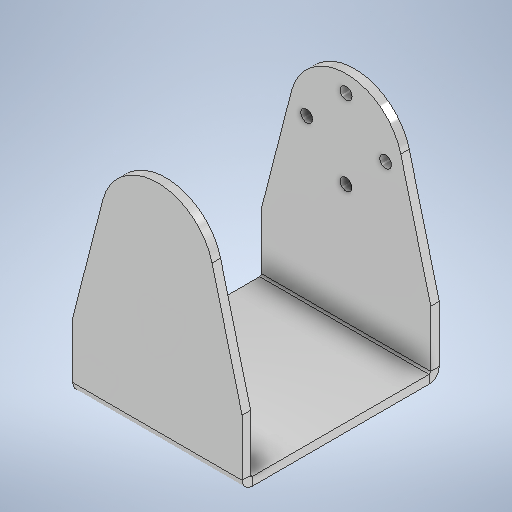
# Autodesk Inventor part: axis_12_bottom_frame(top)
Saved by Autodesk Inventor 2025.2 (Build 292293000, 293)
## iProperties
Created: 2025-05-04
Part Number: axis_12_bottom_frame(top)
Material: Aluminum 6061-AHC
Document SubType Name: Sheet Metal
Designer: User
Density: 2.7 g/cm^3
Sheet Metal Rule: Default_mm
Appearance: Aluminum - Dark
Author: User
Autodesk Inventor part; units mm, degrees
ref_plane "YZ Plane" through (0, 0, 0) normal (1, 0, 0) x (0, 1, 0)
ref_plane "XZ Plane" through (0, 0, 0) normal (0, 1, 0) x (-1, 0, 0)
ref_plane "XY Plane" through (0, 0, 0) normal (0, 0, 1) x (1, 0, 0)
sketch "Sketch1" plane through (0, 0, 0) normal (0, 1, 0) x (-1, 0, 0)
  line L0 (15, -15.965) -> (-15, -15.965)
  line L1 (-15, -15.965) -> (-15, 15.965)
  line L2 (-15, 15.965) -> (15, 15.965)
  line L3 (15, 15.965) -> (15, -15.965)
  point P0 (0, 0)
  dimension "d0" = 30
  dimension "d1" = 15
  dimension "d2" = 31.93
  dimension "d3" = 15.965
  measures "d0" distance of L0.start L0.end
  measures "d1" distance from line of point (0, 0) L3
  measures "d2" distance of L0.end L1.end
  measures "d3" distance from line of point (0, 0) L0
extrude "Plate1" add sketch "Sketch1" along normal blind 1.5
sketch "Sketch2" plane through (15, 0, 17.465) normal (0, 0, -1) x (-1, 0, 0)
  line L0 (30, 0) -> (0, 0)
  line L1 (0, 0) -> (0, 40)
  line L2 (0, 40) -> (30, 40)
  line L3 (30, 40) -> (30, 0)
  constraints: 8 end point
edge flange "Flange1" height 40 angle 90 thickness 1.5 bend radius 0.31 thickness toward (0, 0, -1) relief straight relief width 1.5 relief depth 0.75 edges at (0, 1.5, 15.965) wall of the first edge with corners at (-15, 0, 17.465) (15, 0, 17.465) (15, 40, 17.465) (-15, 40, 17.465)
bend "Bend1"
corner "Corner1"
sketch "Sketch3" plane through (-15, 0, -17.465) normal (0, 0, 1) x (1, 0, 0)
  line L0 (30, 0) -> (0, 0)
  line L1 (0, 0) -> (0, 40)
  line L2 (0, 40) -> (30, 40)
  line L3 (30, 40) -> (30, 0)
  constraints: 8 end point
edge flange "Flange2" height 40 angle 90 thickness 1.5 bend radius 0.31 thickness toward (0, 0, 1) relief straight relief width 1.5 relief depth 0.75 edges at (0, 1.5, -15.965) wall of the first edge with corners at (15, 0, -17.465) (-15, 0, -17.465) (-15, 40, -17.465) (15, 40, -17.465)
bend "Bend2"
corner "Corner2"
sketch "Sketch4" plane through (-15, 40, 17.465) normal (0, 0, 1) x (1, 0, 0)
  circle A0 centre (15, -10) radius 10
  line L0 (0, 0) -> (30, 0) projected
  line L1 (30, 0) -> (30, -38.19) projected
  line L2 (5.3148, -7.5108) -> (0, -28.19)
  line L3 (0, -28.19) -> (0, -38.19)
  line L4 (0, -38.19) -> (30, -38.19)
  line L5 (30, -38.19) -> (30, -28.19)
  line L6 (30, -28.19) -> (24.6852, -7.5108)
  line L7 (0, -38.19) -> (30, -38.19) projected
  line L8 (0, -38.19) -> (0, 0) projected
  point P0 (15, -40)
  point P1 (0, -28.19)
  point P2 (15, 0)
  point P3 (30, -28.19)
  dimension "d25" = 10
  dimension "d26" = 15
  dimension "d27" = 20
  dimension "d29" = 30
  dimension "d30" = 0
  dimension "d31" = 10
  dimension "d32" = 10
  dimension "d33" = 0
  constraints: 10 end point, 2 perpendicular, 2 point on circle, 2 tangent, 1 centre point, 1 collinear, 1 horizontal
  measures "d25" distance from line of A0.centre L0
  measures "d26" distance from line of L1 A0.centre
  measures "d27" diameter of A0
  measures "d29" distance of L3.end L4.end
  measures "d30" distance between parallel lines of L7 L4
  measures "d31" distance of L4.end L5.end
  measures "d32" distance of L2.end L3.end
  measures "d33" distance between parallel lines of L8 L3
extrude "Extrusion1" cut sketch "Sketch4" against normal blind 50 contours A0 L0 L1 L6 | L2 L8 L0 A0
sketch "Sketch5" plane through (15, 1.81, -17.465) normal (0, 0, -1) x (-1, 0, 0)
  arc A0 (24.6852, 30.6792) -> (5.3148, 30.6792) centre (15, 28.19) ccw projected
  circle A1 centre (15, 35.19) radius 1.05
  circle A2 centre (8, 28.19) radius 1.05
  circle A3 centre (15, 21.19) radius 1.05
  circle A4 centre (22, 28.19) radius 1.05
  point P0 (15, -1.81)
  dimension "d36" = 7
  dimension "d37" = 0
  dimension "d38" = 2.1
  dimension "d41" = 360
  constraints: 4 centre point, 9 other
  measures "d36" distance of A0.centre A1.centre
  measures "d37" horizontal distance of A0.centre A1.centre
  measures "d38" diameter of A1
hole "Hole1" at (7, 30, -17.465) at (0, 23, -17.465) at (-7, 30, -17.465) at (0, 37, -17.465) direction (0, 0, 1) diameter 2.1 depth 1.5
equation "\"d48\" = Thickness"
equation "\"d4\" = Thickness"
equation "\"d5\" = BendReliefWidth"
equation "\"d6\" = BendReliefDepth"
equation "\"d7\" = MinimumRemnant"
equation "\"d8\" = TransitionRadius"
equation "\"d11\" = BendRadius"
equation "\"d12\" = CornerReliefSize"
equation "\"d13\" = GapSize"
equation "\"d14\" = JacobiRadiusSize"
equation "\"d15\" = BendReliefWidth"
equation "\"d16\" = BendReliefDepth"
equation "\"d17\" = MinimumRemnant"
equation "\"d18\" = TransitionRadius"
equation "\"d21\" = BendRadius"
equation "\"d22\" = CornerReliefSize"
equation "\"d23\" = GapSize"
equation "\"d24\" = JacobiRadiusSize"
equation "\"BendReliefWidth\" = Thickness"
equation "\"BendReliefDepth\" = 0.5 * Thickness"
equation "\"CornerReliefSize\" = 4 * Thickness"
equation "\"MinimumRemnant\" = 2 * Thickness"
equation "\"TransitionRadius\" = BendRadius"
equation "\"JacobiRadiusSize\" = BendRadius"
equation "\"GapSize\" = Thickness"
equation "\"Thickness\" = 1.5"
equation "\"BendRadius\" = 0.31"
body "Solid1"
